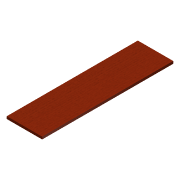
# Autodesk Inventor part: End Plywood Ramp 375
Saved by Autodesk Inventor 2015 (Build 190159000, 159)
## iProperties
Created: 2015-01-20
Part Number: End Plywood Ramp 375
Material: Wood (Oak)
Document SubType Name: Modeling
Designer: Peter
Density: 0.76 g/cm^3
Appearance: White Oak - Natural Medium Gloss
Author: Peter
Autodesk Inventor part; units mm, degrees
ref_plane "YZ Plane" through (0, 0, 0) normal (1, 0, 0) x (0, 1, 0)
ref_plane "XZ Plane" through (0, 0, 0) normal (0, 1, 0) x (-1, 0, 0)
ref_plane "XY Plane" through (0, 0, 0) normal (0, 0, 1) x (1, 0, 0)
sketch "Sketch1" plane through (0, 0, 0) normal (0, 0, 1) x (1, 0, 0)
  line L0 (0, 0) -> (137.16, 0)
  line L1 (137.16, 0) -> (137.16, 9.525)
  line L2 (137.16, 9.525) -> (0, 9.525)
  line L3 (0, 9.525) -> (0, 0)
  dimension "d0" = 9.525
  dimension "d1" = 137.16
  constraints: 8 end point, 2 parallel, 1 horizontal, 1 perpendicular
  measures "d0" distance of L2.end L0.start
  measures "d1" distance of L1.end L2.end
extrude "Extrusion1" add sketch "Sketch1" along normal blind 508
body "Solid1"
